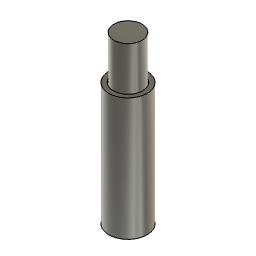
holder (Autodesk Fusion 360 design; units mm, degrees)
Autodesk Fusion 360 part; units mm, degrees
sketch "Sketch1" plane through (0, 0, 0) normal (0, 0, 1) x (1, 0, 0)
  circle A0 centre (0, 0) radius 15
  circle A1 centre (0, 0) radius 13
  circle A2 centre (0, 0) radius 10
  circle A3 centre (0, 0) radius 11.5
  dimension "d1" = 30
  dimension "d2" = 2
  dimension "d3" = 20
  dimension "d5" = 1.5
  constraint coincident A0.centre A1.centre
  constraint concentric A0 A1
  constraint concentric A0 A3
  measures "d1" diameter of A0
  measures "d2" distance of A0 A1
  measures "d3" diameter of A2
  measures "d5" distance of A2 A3
extrude "Extrude1" add sketch "Sketch1" along normal blind 5 contours A0 | A1 | A2 | A3 makes body 1
extrude "Extrude2" add sketch "Sketch1" along normal blind 96 contours A0 bodies 1
ref_plane "WorkPlane2" through (0, 0, 43) normal (0, 0, 1) x (1, 0, 0)
sketch "Sketch3" plane through (0, 0, 43) normal (0, 0, 1) x (1, 0, 0)
  circle A0 centre (0, 0) radius 12
  dimension "d12" = 24
  constraint coincident A0.centre origin
  measures "d12" diameter of A0
sketch "Sketch4" plane through (0, 0, 43) normal (0, 0, 1) x (1, 0, 0)
extrude "Extrude3" add sketch "Sketch3" along normal blind 44 separate body makes body 2
sketch "Sketch5" plane through (0, 0, 96) normal (0, 0, 1) x (-1, 0, 0)
  circle A0 centre (0, 0) radius 13
  circle A1 centre (0, 0) radius 15
  circle A2 centre (0, 0) radius 15
  constraint concentric A0 A2
extrude "Extrude4" add sketch "Sketch5" against normal blind 2 contours A0 | A1 A2 bodies 1
sketch "Sketch6" plane through (0, 0, 96) normal (0, 0, 1) x (-1, 0, 0)
  circle A0 centre (0, 0) radius 15
  circle A1 centre (0, 0) radius 11.5
  dimension "d17" = 23
  constraint coincident A0.centre A1.centre
  measures "d17" diameter of A1
extrude "Extrude5" cut sketch "Sketch6" against normal blind 3 contours A1 bodies 1
sketch "Sketch7" plane through (0, 0, 87) normal (0, 0, 1) x (-1, 0, 0)
  circle A0 centre (0, 0) radius 12
  circle A1 centre (0, 0) radius 11
  dimension "d22" = 22
  constraint coincident A0.centre A1.centre
  measures "d22" diameter of A1
extrude "Extrude6" add sketch "Sketch7" along normal blind 43 contours A1 bodies 2
